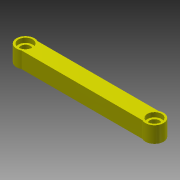
# Autodesk Inventor part: ARM
Saved by Autodesk Inventor 2013 (Build 170138000, 138)
## iProperties
Created: 2013-11-16
Part Number: ARM
Material: Generic
Document SubType Name: Modeling
Designer: employee
Density: 1 g/cm^3
Author: employee
Autodesk Inventor part; units mm, degrees
ref_plane "YZ Plane" through (0, 0, 0) normal (1, 0, 0) x (0, 1, 0)
ref_plane "XZ Plane" through (0, 0, 0) normal (0, 1, 0) x (-1, 0, 0)
ref_plane "XY Plane" through (0, 0, 0) normal (0, 0, 1) x (1, 0, 0)
sketch "Sketch1" plane through (0, 0, 0) normal (0, 0, 1) x (1, 0, 0)
  arc A0 (6.3048, 12.5) -> (6.3048, -12.5) centre (0, 0) ccw
  arc A1 (193.6952, -12.5) -> (193.6952, 12.5) centre (200, 0) ccw
  line L0 (6.3048, 12.5) -> (193.6952, 12.5)
  line L1 (193.6952, -12.5) -> (6.3048, -12.5)
  dimension "d0" = 25
  dimension "d2" = 14
  dimension "d3" = 200
  constraints: 4 end point, 4 point on circle, 2 centre point, 2 parallel, 1 coincident, 1 equal radius, 1 horizontal, 1 horizontal alignment
  measures "d0" distance between parallel lines of L0 L1
  measures "d2" radius of A0
  measures "d3" distance of point (0, 0) A1.centre
extrude "Extrusion1" add sketch "Sketch1" along normal blind 25
sketch "Sketch2" plane through (0, 0, 25) normal (0, 0, 1) x (1, 0, 0)
  arc A0 (6.3048, 12.5) -> (6.3048, -12.5) centre (0, 0) ccw projected
  arc A1 (193.6952, -12.5) -> (193.6952, 12.5) centre (200, 0) ccw projected
  circle A2 centre (0, 0) radius 11.05
  circle A3 centre (200, 0) radius 11.05
  dimension "d6" = 22.1
  constraints: 2 centre point, 2 coincident, 1 equal radius
  measures "d6" diameter of A2
extrude "Extrusion2" cut sketch "Sketch2" against normal blind 7
sketch "Sketch3" plane through (0, 0, 0) normal (0, 0, -1) x (-1, 0, 0)
  circle A0 centre (-200, 0) radius 11.05 projected
  circle A1 centre (0, 0) radius 11.05 projected
extrude "Extrusion3" cut sketch "Sketch3" against normal blind 7
sketch "Sketch4" plane through (200, 0, 7) normal (0, 0, -1) x (-1, 0, 0)
  circle A0 centre (0, 0) radius 11.05 projected
  circle A1 centre (200, 0) radius 11.05 projected
  circle A2 centre (0, 0) radius 7.55
  circle A3 centre (200, 0) radius 7.55
  dimension "d12" = 15.1
  constraints: 2 centre point, 2 coincident, 1 equal radius
  measures "d12" diameter of A3
extrude "Extrusion4" cut sketch "Sketch4" against normal through all contours A2 | A3
chamfer "Chamfer1" distance 3.5 angle 45 2 edges at (207.55, 0, 7) (7.55, 0, 7)
body "Solid1"
